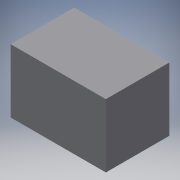
# Autodesk Inventor part: Generator
Saved by Autodesk Inventor 2019 (Build 230136000, 136)
## iProperties
Created: 2019-12-03
Part Number: Generator
Material: Generic
Document SubType Name: Modeling
Designer: Administrator
Density: 1 g/cm^3
Appearance: Default
Author: Administrator
Autodesk Inventor part; units mm, degrees
ref_plane "YZ Plane" through (0, 0, 0) normal (1, 0, 0) x (0, 1, 0)
ref_plane "XZ Plane" through (0, 0, 0) normal (0, 1, 0) x (-1, 0, 0)
ref_plane "XY Plane" through (0, 0, 0) normal (0, 0, 1) x (1, 0, 0)
sketch "Sketch1" plane through (0, 0, 0) normal (0, 1, 0) x (-1, 0, 0)
  line L0 (-381, 254) -> (381, 254)
  line L1 (381, 254) -> (381, -254)
  line L2 (381, -254) -> (-381, -254)
  line L3 (-381, -254) -> (-381, 254)
  line L4 (-381, 254) -> (381, -254) construction
  line L5 (381, 254) -> (-381, -254) construction
  point P0 (0, 0)
  dimension "d0" = 762
  dimension "d1" = 508
  constraints: 12 end point, 2 midpoint, 2 parallel, 1 horizontal, 1 perpendicular
  measures "d0" distance of L1.end L2.end
  measures "d1" distance of L0.end L1.end
extrude "Extrusion1" add sketch "Sketch1" along normal blind 508
sketch "Sketch2" plane through (381, 0, -254) normal (0, 0, -1) x (-1, 0, 0)
  line L0 (0, 0) -> (0, 508) projected
  line L1 (0, 254) -> (127, 254) construction
  circle A0 centre (127, 254) radius 9.525
  circle A1 centre (127, 254) radius 12.7
  point P0 (381, 0)
  dimension "d4" = 127
  dimension "d5" = 19.05
  dimension "d6" = 25.4
  constraints: 2 centre point, 2 coincident, 2 end point, 1 horizontal, 1 midpoint
  measures "d4" distance of L1.start L1.end
  measures "d5" diameter of A0
  measures "d6" diameter of A1
extrude "Extrusion2" add sketch "Sketch2" along normal blind 2.54
body "Solid1"
